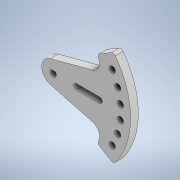
# Autodesk Inventor part: ParallelMecha_Capstondisc_V3
Saved by Autodesk Inventor 2022 (Build 260153000, 153)
## iProperties
Created: 2022-08-01
Part Number: ParallelMecha_Capstondisc_V3
Material: Generisch
Document SubType Name: Modeling
Designer: alexw
Density: 1 g/cm^3
Appearance: Vorgabe
Author: alexw
Autodesk Inventor part; units mm, degrees
ref_plane "YZ Plane" through (0, 0, 0) normal (1, 0, 0) x (0, 1, 0)
ref_plane "XZ Plane" through (0, 0, 0) normal (0, 1, 0) x (-1, 0, 0)
ref_plane "XY Plane" through (0, 0, 0) normal (0, 0, 1) x (1, 0, 0)
sketch "Skizze1" plane through (0, 0, 0) normal (0, 0, 1) x (1, 0, 0)
  circle A0 centre (0, 0) radius 15
  circle A1 centre (0, 0) radius 4
  line L0 (0, 0) -> (15, 0) construction
  line L1 (-7.5, 12.9904) -> (78.1227, 62.4247) construction
  line L2 (-7.5, -12.9904) -> (78.1227, -62.4247) construction
  line L3 (78.1227, 62.4247) -> (78.1227, -62.4247) construction
  arc A2 (78.1227, -62.4247) -> (78.1227, 62.4247) centre (0, 0) ccw
  arc A3 (56.1396, -49.7327) -> (56.1396, 49.7327) centre (0, 0) ccw
  line L4 (56.1396, 49.7327) -> (78.1227, 62.4247)
  line L5 (56.1396, -49.7327) -> (78.1227, -62.4247)
  arc A4 (51.0992, 29.2211) -> (57.1349, 48.586) centre (47.9933, 40.8122) ccw
  line L6 (-3.8823, 14.4889) -> (51.0992, 29.2211)
  line L7 (-3.8823, -14.4889) -> (51.0992, -29.2211)
  arc A5 (57.1349, -48.586) -> (51.0992, -29.2211) centre (47.9933, -40.8122) ccw
  line L8 (30, 0) -> (60, 0) construction
  line L9 (30, 3.5) -> (60, 3.5)
  line L10 (60, -3.5) -> (30, -3.5)
  arc A6 (30, 3.5) -> (30, -3.5) centre (30, 0) ccw
  arc A7 (60, -3.5) -> (60, 3.5) centre (60, 0) ccw
  line L11 (0, 0) -> (78.1227, 0) construction
  arc A8 (67.1312, -56.0787) -> (67.1312, 56.0787) centre (0, 0) ccw construction
  circle A9 centre (76.5051, 42.4074) radius 4
  line L12 (76.5051, 42.4074) -> (0, 0) construction
  circle A10 centre (83.4697, 26.1578) radius 4
  circle A11 centre (87.0246, 8.8396) radius 4
  circle A12 centre (87.0246, -8.8396) radius 4
  circle A13 centre (83.4697, -26.1578) radius 4
  circle A14 centre (76.5051, -42.4074) radius 4
  line L13 (2.6458, 3) -> (-2.6458, 3)
  point P0 (75, 0)
  point P1 (45, 0)
  dimension "d0" = 8
  dimension "d1" = 30
  dimension "d2" = 30
  dimension "d3" = 100
  dimension "d4" = 25
  dimension "d5" = 12
  dimension "d6" = 15
  dimension "d7" = 12
  dimension "d8" = 15
  dimension "d10" = 60
  dimension "d13" = 0
  dimension "d14" = 30
  dimension "d15" = 7
  dimension "d16" = 30
  dimension "d27" = 8
  dimension "d28" = 60
  dimension "d29" = 1
  dimension "d32" = 58
  dimension "d35" = 3
  constraints: 30 end point, 25 point on circle, 15 centre point, 12 tangent, 4 midpoint, 3 coincident, 3 concentric, 2 collinear, 2 horizontal, 2 point on line, 1 equal length, 1 parallel, 1 vertical, 11 other
  measures "d0" diameter of A1
  measures "d1" diameter of A0
  measures "d2" angle of L1 L0
  measures "d3" radius of A2
  measures "d4" radial gap between concentric circles of A2 A3
  measures "d5" radius of A4
  measures "d6" angle of L0 L6
  measures "d7" radius of A5
  measures "d8" angle of L0 L7
  measures "d10" distance of point (75, 0) point (15, 0)
  measures "d13" distance between parallel lines of L8 L0
  measures "d14" distance of L0.end point (45, 0)
  measures "d15" distance between parallel lines of L10 L9
  measures "d16" distance of L8.start L8.end
  measures "d27" diameter of A9
  measures "d28" angle of L1 L2
  measures "d29" angle of L1 L12
  measures "d35" distance from line of L13 L0.start
extrude "Extrusion1" add sketch "Skizze1" along normal blind 10 contours A0 | A0 L6 A4 A3 A5 L7 | A3 L4 A2 L5 | L13 A1 picked at (-0.6179, 3.1815)
fillet "Rundung1" radius 4 4 edges at (78.1227, 62.4247, 5) (78.1227, -62.4247, 5) (56.1396, 49.7327, 5) (56.1396, -49.7327, 5)
equation "\"d7\" = d5"
equation "\"d8\" = d6"
equation "\"d14\" = 0.5 * d10"
equation "\"d32\" = d28 - 2 * d29"
